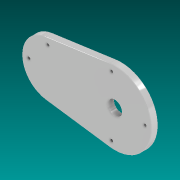
# Autodesk Inventor part: onderkantBase
Saved by Autodesk Inventor 2020.2 (Build 242310000, 310)
## iProperties
Created: 2020-05-15
Part Number: onderkantBase
Material: Aluminum 6061
Document SubType Name: Modeling
Designer: Svend
Density: 2.7 g/cm^3
Appearance: Aluminum - Polished
Author: Svend
Autodesk Inventor part; units mm, degrees
ref_plane "YZ Plane" through (0, 0, 0) normal (1, 0, 0) x (0, 1, 0)
ref_plane "XZ Plane" through (0, 0, 0) normal (0, 1, 0) x (-1, 0, 0)
ref_plane "XY Plane" through (0, 0, 0) normal (0, 0, 1) x (1, 0, 0)
sketch "Sketch1" plane through (0, 0, 0) normal (0, 0, 1) x (1, 0, 0)
  arc A0 (-5.9149, 42.0864) -> (-5.9149, -42.0864) centre (0, 0) ccw
  arc A1 (92.2885, -55.888) -> (92.2885, 55.888) centre (100.143, 0) ccw
  line L0 (-42.5, 0) -> (156.5802, 0)
  line L1 (92.2885, 55.888) -> (-5.9149, 42.0864)
  line L2 (-5.9149, -42.0864) -> (92.2885, -55.888)
  line L3 (-3.1314, 22.281) -> (95.0719, 36.0826)
  arc A2 (95.0719, -36.0826) -> (95.0719, 36.0826) centre (100.143, 0) ccw
  line L4 (95.0719, -36.0826) -> (-3.1314, -22.281)
  arc A3 (-3.1314, 22.281) -> (-3.1314, -22.281) centre (0, 0) ccw
  circle A4 centre (100.143, 0) radius 11
  point P0 (146.5802, 0)
  point P1 (95.0719, 46.1809)
  point P2 (95.0719, -46.1809)
  point P3 (-32.5, 0)
  point P4 (-3.1314, 32.3793)
  point P5 (-3.1314, -32.3793)
  dimension "d0" = 85
  dimension "d1" = 100.143
  dimension "d2" = 8
  dimension "d3" = 20
  dimension "d4" = 10
  dimension "d5" = 10
  dimension "d6" = 10
  dimension "d7" = 10
  dimension "d8" = 10
  dimension "d9" = 10
  dimension "d22" = 22
  constraints: 10 end point, 10 point on circle, 5 centre point, 4 tangent, 4 vertical alignment, 3 point on line, 2 coincident, 2 horizontal alignment, 1 horizontal, 3 other
  measures "d0" diameter of A0
  measures "d1" distance of A0.centre A1.centre
  measures "d2" angle of L0 L1
  measures "d3" distance between parallel lines of L1 L3
  measures "d4" distance from line of point (-3.131, -32.379) L4
  measures "d5" distance of L0.end point (146.58, 0)
  measures "d6" distance from line of L3 point (95.072, 46.181)
  measures "d7" distance from line of L3 point (-3.131, 32.379)
  measures "d8" distance from line of point (95.072, -46.181) L4
  measures "d9" distance of L0.start point (-32.5, 0)
  measures "d22" diameter of A4
extrude "Extrusion1" add sketch "Sketch1" along normal blind 10 contours L1 A1 L0 A2 L3 A3 A0 | L0 A3 L4 A2 A1 L2 A0 | A3 L3 A2 L0 A4 | L0 A4 A2 L4 A3
hole "Hole1" at (-32.5, 0, 0) at (-3.1314, 32.3793, 0) at (95.0719, 46.1809, 0) at (146.5802, 0, 0) at (95.0719, -46.1809, 0) direction (0, 0, 1) diameter 4.134 end through all thread size "M5x0.8" class "6H" standard "ISO Metric profile"
chamfer "Chamfer2" distance 0.5 angle 45 20 edges at (43.1868, -48.9872, 10) (156.5802, 0, 10) (43.1868, 48.9872, 10) (-42.5, 0, 10) (43.1868, -48.9872, 0) (156.5802, 0, 0) (43.1868, 48.9872, 0) (-42.5, 0, 0) (95.0719, -48.2479, 0) (95.0719, -48.2479, 10) (95.0719, 44.1139, 0) (95.0719, 44.1139, 10) (-3.1314, 30.3123, 0) (-3.1314, 30.3123, 10) (-32.5, -2.067, 0) (-32.5, -2.067, 10) (89.143, 0, 10) (89.143, 0, 0) (146.5802, -2.067, 0) (146.5802, -2.067, 10)
equation "\"d4\" = 0.5 * d3"
equation "\"d5\" = 0.5 * d3"
equation "\"d6\" = 0.5 * d3"
equation "\"d7\" = 0.5 * d3"
equation "\"d8\" = d6"
equation "\"d9\" = d7"
body "Solid1"
